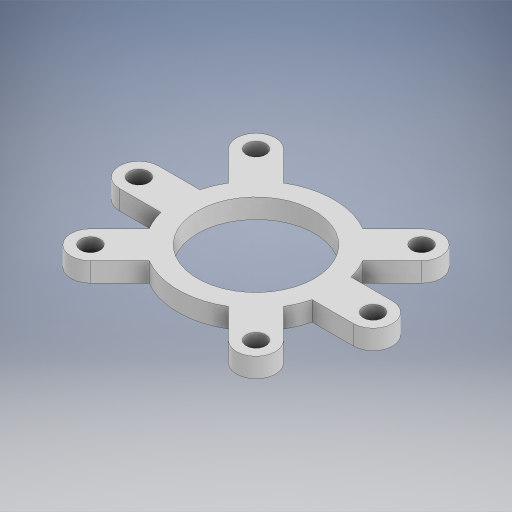
# Autodesk Inventor part: CE-1.3.1
Saved by Autodesk Inventor 2024 (Build 280153000, 153)
## iProperties
Created: 2024-01-25
Part Number: CE-1.3.1
Material: Generic
Document SubType Name: Modeling
Designer: Alex
Density: 1 g/cm^3
Appearance: Default
Author: Alex
Autodesk Inventor part; units mm, degrees
ref_plane "YZ Plane" through (0, 0, 0) normal (1, 0, 0) x (0, 1, 0)
ref_plane "XZ Plane" through (0, 0, 0) normal (0, 1, 0) x (-1, 0, 0)
ref_plane "XY Plane" through (0, 0, 0) normal (0, 0, 1) x (1, 0, 0)
sketch "Sketch1" plane through (0, 0, 0) normal (0, 1, 0) x (-1, 0, 0)
  circle A0 centre (0, 0) radius 60 construction
  circle A1 centre (0, 0) radius 30
  circle A2 centre (60, 0) radius 5
  arc A3 (59.1667, -9.9652) -> (59.1667, 9.9652) centre (60, 0) ccw
  line L0 (60, -10) -> (38.7298, -10)
  line L1 (60, 10) -> (38.7298, 10)
  circle A4 centre (42.4264, 42.4264) radius 5
  arc A5 (48.8836, 34.7907) -> (34.7907, 48.8836) centre (42.4264, 42.4264) ccw
  line L2 (49.4975, 35.3553) -> (34.4572, 20.3151)
  line L3 (35.3553, 49.4975) -> (20.3151, 34.4572)
  circle A6 centre (0, 60) radius 5
  arc A7 (9.9652, 59.1667) -> (-9.9652, 59.1667) centre (0, 60) ccw
  line L4 (10, 60) -> (10, 38.7298)
  line L5 (-10, 60) -> (-10, 38.7298)
  circle A8 centre (-42.4264, 42.4264) radius 5
  arc A9 (-34.7907, 48.8836) -> (-48.8836, 34.7907) centre (-42.4264, 42.4264) ccw
  line L6 (-35.3553, 49.4975) -> (-20.3151, 34.4572)
  line L7 (-49.4975, 35.3553) -> (-34.4572, 20.3151)
  circle A10 centre (-60, 0) radius 5
  arc A11 (-59.1667, 9.9652) -> (-59.1667, -9.9652) centre (-60, 0) ccw
  line L8 (-60, 10) -> (-38.7298, 10)
  line L9 (-60, -10) -> (-38.7298, -10)
  circle A12 centre (-42.4264, -42.4264) radius 5
  arc A13 (-48.8836, -34.7907) -> (-34.7907, -48.8836) centre (-42.4264, -42.4264) ccw
  line L10 (-49.4975, -35.3553) -> (-34.4572, -20.3151)
  line L11 (-35.3553, -49.4975) -> (-20.3151, -34.4572)
  circle A14 centre (0, -60) radius 5
  arc A15 (-9.9652, -59.1667) -> (9.9652, -59.1667) centre (0, -60) ccw
  line L12 (-10, -60) -> (-10, -38.7298)
  line L13 (10, -60) -> (10, -38.7298)
  circle A16 centre (42.4264, -42.4264) radius 5
  arc A17 (34.7907, -48.8836) -> (48.8836, -34.7907) centre (42.4264, -42.4264) ccw
  line L14 (35.3553, -49.4975) -> (20.3151, -34.4572)
  line L15 (49.4975, -35.3553) -> (34.4572, -20.3151)
  arc A18 (34.4572, -20.3151) -> (38.7298, -10) centre (0, 0) ccw
  arc A19 (-20.3151, -34.4572) -> (20.3151, -34.4572) centre (0, 0) ccw
  arc A20 (-38.7298, -10) -> (-34.4572, -20.3151) centre (0, 0) ccw
  arc A21 (-34.4572, 20.3151) -> (-38.7298, 10) centre (0, 0) ccw
  arc A22 (38.7298, 10) -> (34.4572, 20.3151) centre (0, 0) ccw
  arc A23 (20.3151, 34.4572) -> (-20.3151, 34.4572) centre (0, 0) ccw
  circle A24 centre (0, 0) radius 40 construction
  dimension "d0" = 120
  dimension "d1" = 60
  dimension "d3" = 10
  dimension "d4" = 20
  dimension "d5" = 10
  dimension "d8" = 360
  dimension "d10" = 40
  constraints: 47 point on circle, 32 end point, 24 centre point, 12 coincident, 2 tangent, 1 horizontal, 1 parallel, 100 other
  measures "d0" diameter of A0
  measures "d1" diameter of A1
  measures "d3" diameter of A2
  measures "d4" diameter of A3
  measures "d5" distance from line of point (0, 0) L1
  measures "d10" radius of A23
extrude "Extrusion1" add sketch "Sketch1" along normal blind 10 contours L0 A18 L15 A17 L14 A19 L11 A13 L10 A20 L9 A11 L8 A21 L7 A9 L6 A23 L3 A5 L2 A22 L1 A3
body "Solid1"
